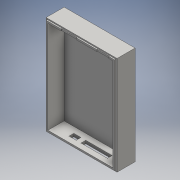
# Autodesk Inventor part: Arduino_Box_Upper
Saved by Autodesk Inventor 2016 (Build 200138000, 138)
## iProperties
Created: 2016-07-06
Part Number: Arduino_Box_Upper
Material: Generic
Document SubType Name: Modeling
Designer: jorge
Density: 1 g/cm^3
Appearance: Default
Author: jorge
Autodesk Inventor part; units mm, degrees
ref_plane "YZ Plane" through (0, 0, 0) normal (1, 0, 0) x (0, 1, 0)
ref_plane "XZ Plane" through (0, 0, 0) normal (0, 1, 0) x (-1, 0, 0)
sketch "Sketch1" plane through (0, 0, 0) normal (0, 1, 0) x (-1, 0, 0)
  line L0 (0, 0) -> (59, 0)
  line L1 (59, 0) -> (59, -82)
  line L2 (59, -82) -> (0, -82)
  line L3 (0, -82) -> (0, 0)
  dimension "d0" = 82
  dimension "d1" = 59
  constraints: 8 end point, 2 parallel, 1 horizontal, 1 perpendicular
  measures "d0" distance of L0.end L1.end
  measures "d1" distance of L1.end L2.end
extrude "Extrusion1" add sketch "Sketch1" along normal blind 32
ref_plane "Work Plane1" through (0, 2.5, 0) normal (0, -1, 0) x (1, 0, 0)
sketch "Sketch2" plane through (0, 2.5, 0) normal (0, -1, 0) x (1, 0, 0)
  line L0 (-2.5, -2.5) -> (-56.5, -2.5)
  line L1 (-56.5, -2.5) -> (-56.5, -79.5)
  line L2 (-56.5, -79.5) -> (-2.5, -79.5)
  line L3 (-2.5, -79.5) -> (-2.5, -2.5)
  line L4 (0, 0) -> (0, -82) projected
  line L5 (-59, 0) -> (0, 0) projected
  line L6 (-59, -82) -> (-59, 0) projected
  line L7 (0, -82) -> (-59, -82) projected
  dimension "d5" = 2.5
  dimension "d6" = 2.5
  dimension "d7" = 2.5
  dimension "d8" = 2.5
  constraints: 8 end point, 2 parallel, 1 horizontal, 1 perpendicular
  measures "d5" distance between parallel lines of L4 L3
  measures "d6" distance between parallel lines of L5 L0
  measures "d7" distance between parallel lines of L6 L1
  measures "d8" distance between parallel lines of L7 L2
extrude "Extrusion2" cut sketch "Sketch2" against normal blind 27 contours L3 L2 L1 L0
sketch "Sketch3" plane through (0, 2.5, 0) normal (0, -1, 0) x (1, 0, 0)
  line L0 (-3, -3) -> (-56, -3) construction
  line L1 (-56, -3) -> (-56, -79) construction
  line L2 (-56, -79) -> (-3, -79) construction
  line L3 (-3, -79) -> (-3, -3) construction
  line L4 (-2.5, -2.5) -> (-2.5, -79.5) projected
  line L5 (-56.5, -2.5) -> (-2.5, -2.5) projected
  line L6 (-56.5, -79.5) -> (-56.5, -2.5) projected
  line L7 (-2.5, -79.5) -> (-56.5, -79.5) projected
  circle A0 centre (-53.8, -24.59) radius 1.65
  circle A1 centre (-5.54, -23.32) radius 1.65
  circle A2 centre (-38.56, -75.39) radius 1.65
  circle A3 centre (-10.62, -75.39) radius 1.65
  point P0 (0, 0)
  dimension "d11" = 0.5
  dimension "d12" = 0.5
  dimension "d13" = 0.5
  dimension "d14" = 0.5
  dimension "d15" = 3.3
  dimension "d16" = 20.32
  dimension "d17" = 2.54
  dimension "d18" = 7.62
  dimension "d19" = 72.39
  dimension "d20" = 21.59
  dimension "d22" = 50.8
  dimension "d23" = 35.56
  dimension "d24" = 72.39
  constraints: 8 end point, 4 centre point, 3 equal radius, 2 parallel, 1 horizontal, 1 perpendicular
  measures "d11" distance between parallel lines of L4 L3
  measures "d12" distance between parallel lines of L5 L0
  measures "d13" distance between parallel lines of L6 L1
  measures "d14" distance between parallel lines of L7 L2
  measures "d15" diameter of A0
  measures "d16" distance from line of A1.centre L0
  measures "d17" distance from line of L3 A1.centre
  measures "d18" distance from line of L3 A3.centre
  measures "d19" distance from line of L0 A3.centre
  measures "d20" distance from line of L0 A0.centre
  measures "d22" distance from line of L3 A0.centre
  measures "d23" distance from line of L3 A2.centre
  measures "d24" distance from line of L0 A2.centre
extrude "Extrusion3" cut sketch "Sketch3" along normal blind 27 contours A0 | A1 | A2 | A3
sketch "Sketch4" plane through (-59, 0, 0) normal (0, 0, 1) x (1, 0, 0)
  line L0 (13.4, 5.6) -> (26.4, 5.6)
  line L1 (26.4, 5.6) -> (26.4, 16.5)
  line L2 (26.4, 16.5) -> (13.4, 16.5)
  line L3 (13.4, 16.5) -> (13.4, 5.6)
  line L4 (43.3, 5.6) -> (53.2, 5.6)
  line L5 (53.2, 5.6) -> (53.2, 16.5)
  line L6 (53.2, 16.5) -> (43.3, 16.5)
  line L7 (43.3, 16.5) -> (43.3, 5.6)
  line L8 (56.5, 2.5) -> (2.5, 2.5) projected
  line L9 (2.5, 2.5) -> (2.5, 29.5) projected
  line L10 (56.5, 2.5) -> (56.5, 29.5) projected
  point P0 (59, 0)
  dimension "d27" = 13
  dimension "d28" = 10.9
  dimension "d29" = 9.9
  dimension "d31" = 14
  dimension "d32" = 10.9
  dimension "d33" = 3.3
  constraints: 16 end point, 4 parallel, 2 collinear, 2 horizontal, 2 perpendicular
  measures "d27" distance of L1.end L2.end
  measures "d28" distance of L2.end L0.start
  measures "d29" distance of L5.end L6.end
  measures "d31" distance between parallel lines of L8 L2
  measures "d32" distance between parallel lines of L9 L3
  measures "d33" distance between parallel lines of L10 L5
extrude "Extrusion4" cut sketch "Sketch4" against normal blind 5
sketch "Sketch5" plane through (0, 0, -82) normal (0, 0, -1) x (-1, 0, 0)
  line L0 (11.5, 24.5) -> (33.5, 24.5)
  line L1 (33.5, 24.5) -> (33.5, 20.5)
  line L2 (33.5, 20.5) -> (11.5, 20.5)
  line L3 (11.5, 20.5) -> (11.5, 24.5)
  line L4 (37.5, 24.5) -> (43.5, 24.5)
  line L5 (43.5, 24.5) -> (43.5, 20.5)
  line L6 (43.5, 20.5) -> (37.5, 20.5)
  line L7 (37.5, 20.5) -> (37.5, 24.5)
  line L8 (56.5, 2.5) -> (2.5, 2.5) projected
  line L9 (2.5, 2.5) -> (2.5, 29.5) projected
  point P0 (0, 0)
  dimension "d36" = 22
  dimension "d37" = 4
  dimension "d38" = 4
  dimension "d39" = 22
  dimension "d40" = 9
  dimension "d41" = 6
  dimension "d42" = 4
  constraints: 16 end point, 4 parallel, 2 horizontal, 2 perpendicular, 1 collinear
  measures "d36" distance of L0.start L0.end
  measures "d37" distance of L0.end L1.end
  measures "d38" distance of L4.end L5.end
  measures "d39" distance between parallel lines of L8 L0
  measures "d40" distance between parallel lines of L9 L3
  measures "d41" distance of L4.start L4.end
  measures "d42" distance between parallel lines of L7 L1
extrude "Extrusion5" cut sketch "Sketch5" against normal blind 5
sketch "Sketch6" plane through (-59, 0, -82) normal (-1, 0, 0) x (0, 0, 1)
  circle A0 centre (57.41, 6) radius 1.6
  line L0 (79.5, 2.5) -> (79.5, 29.5) projected
  line L1 (82, 0) -> (0, 0) projected
  dimension "d45" = 3.2
  dimension "d46" = 22.09
  dimension "d47" = 6
  constraints: 1 centre point
  measures "d45" diameter of A0
  measures "d46" distance from line of A0.centre L0
  measures "d47" distance from line of L1 A0.centre
sketch "Sketch7" plane through (0, 0, 0) normal (1, 0, 0) x (0, 0, -1)
  circle A0 centre (23.32, 6) radius 1.6
  line L0 (82, 0) -> (0, 0) projected
  line L1 (2.5, 2.5) -> (2.5, 29.5) projected
  dimension "d48" = 6
  dimension "d49" = 20.82
  dimension "d50" = 3.2
  constraints: 1 centre point
  measures "d48" distance from line of L0 A0.centre
  measures "d49" distance from line of L1 A0.centre
  measures "d50" diameter of A0
sketch "Sketch8" plane through (0, 0, -82) normal (0, 0, -1) x (-1, 0, 0)
  circle A0 centre (10.62, 6) radius 1.6
  circle A1 centre (38.56, 6) radius 1.6
  line L0 (59, 0) -> (0, 0) projected
  line L1 (2.5, 2.5) -> (2.5, 29.5) projected
  dimension "d51" = 3.2
  dimension "d52" = 3.2
  dimension "d53" = 6
  dimension "d54" = 6
  dimension "d55" = 8.12
  dimension "d56" = 36.06
  constraints: 2 centre point
  measures "d51" diameter of A0
  measures "d52" diameter of A1
  measures "d53" distance from line of L0 A0.centre
  measures "d54" distance from line of L0 A1.centre
  measures "d55" distance from line of L1 A0.centre
  measures "d56" distance from line of L1 A1.centre
extrude "Extrusion6" cut sketch "Sketch6" against normal blind 5
extrude "Extrusion7" cut sketch "Sketch7" against normal blind 5
extrude "Extrusion8" cut sketch "Sketch8" against normal blind 5
sketch "Sketch9" plane through (-59, 0, 0) normal (0, 0, 1) x (1, 0, 0)
  line L0 (-2.1645, 16) -> (66.4826, 16)
  line L1 (59, 0) -> (0, 0) projected
  dimension "d63" = 16
  constraints: 2 end point, 1 horizontal
  measures "d63" distance between parallel lines of L1 L0
split body "Split1" sketch "Sketch9" result one side removed curves L0 removed pieces at (-32.4383, 0.5, -41.3152)
sketch "Sketch10" plane through (-59, 16, -82) normal (0, -1, 0) x (1, 0, 0)
  line L0 (0, 82) -> (59, 82) projected
  line L1 (59, 82) -> (59, 0) projected
  line L2 (0, 82) -> (59, 82)
  line L3 (59, 82) -> (59, 0)
  line L4 (59, 0) -> (0, 0)
  line L5 (0, 0) -> (0, 82)
  line L6 (58, 1) -> (1, 1)
  line L7 (1, 1) -> (1, 81)
  line L8 (1, 81) -> (58, 81)
  line L9 (58, 81) -> (58, 1)
  dimension "d64" = 1
  dimension "d65" = 1
  dimension "d66" = 1
  dimension "d67" = 1
  constraints: 16 end point, 4 parallel, 2 horizontal, 2 perpendicular
  measures "d64" distance between parallel lines of L5 L7
  measures "d65" distance between parallel lines of L1 L9
  measures "d66" distance between parallel lines of L8 L0
  measures "d67" distance between parallel lines of L4 L6
extrude "Extrusion9" cut sketch "Sketch10" against normal blind 1
body "Solid1"
